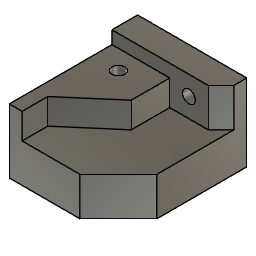
Robocon Task 1-1 (Autodesk Fusion 360 design; units mm, degrees)
Autodesk Fusion 360 part; units mm, degrees
sketch "Sketch1" plane through (0, 0, 0) normal (0, 0, 1) x (1, 0, 0)
  line L0 (0, 0) -> (55, 0)
  line L1 (0, 0) -> (0, 100)
  line L2 (0, 100) -> (85, 100)
  line L3 (85, 100) -> (85, 30)
  line L4 (85, 30) -> (55, 0)
  dimension "d1" = 55
  dimension "d2" = 100
  dimension "d3" = 85
  dimension "d4" = 70
  constraint coincident L0.start L1.start
  constraint horizontal L0
  constraint perpendicular L0 L1
  constraint perpendicular L1 L2
  constraint perpendicular L2 L3
  measures "d1" distance of L0.start L0.end
  measures "d2" distance of L0.start L1.end
  measures "d3" distance of L1.end L2.end
  measures "d4" distance of L2.end L3.end
extrude "Extrude1" add sketch "Sketch1" along normal blind 30
sketch "Sketch2" plane through (0, 0, 30) normal (0, 0, 1) x (-1, 0, 0)
  line L0 (0, 0) -> (-55, 0)
  line L1 (-55, 0) -> (-85, -30)
  line L2 (-85, -30) -> (-85, -100)
  line L3 (-85, -100) -> (0, -100)
  line L4 (0, -100) -> (0, 0)
  line L5 (0, 0) -> (-10, 0)
  line L6 (-10, 0) -> (-10, -20)
  line L7 (0, 0) -> (0, -100)
  line L8 (-85, -100) -> (-85, -90)
  line L9 (-85, -90) -> (-75, -80)
  line L10 (-75, -80) -> (-45, -80)
  line L11 (-45, -80) -> (-45, -50)
  line L12 (-45, -50) -> (-10, -20)
  dimension "d7" = 10
  dimension "d8" = 20
  dimension "d12" = 30
  dimension "d13" = 30
  constraint coincident L0.start L4.end
  constraint perpendicular L4 L5
  constraint perpendicular L5 L6
  constraint coincident L3.end L4.start
  constraint coincident L2.end L3.start
  constraint perpendicular L3 L8
  constraint horizontal L10
  constraint perpendicular L10 L11
  measures "d7" distance of L0.start L5.end
  measures "d8" distance of L5.end L6.end
  measures "d12" distance of L9.end L10.end
  measures "d13" distance of L10.end L11.end
extrude "Extrude2" add sketch "Sketch2" along normal blind 20 contours L0 L2 L3 L4 L5 L6 L7 L8 L9 L10 L11 L12
sketch "Sketch3" plane through (0, 0, 50) normal (0, 0, 1) x (-1, 0, 0)
  line L0 (-85, -100) -> (0, -100)
  line L1 (0, -100) -> (0, 0)
  line L2 (0, 0) -> (-10, 0)
  line L3 (-10, 0) -> (-10, -20)
  line L4 (-10, -20) -> (-45, -50)
  line L5 (-45, -50) -> (-45, -80)
  line L6 (-45, -80) -> (-75, -80)
  line L7 (-75, -80) -> (-85, -90)
  line L8 (-85, -90) -> (-85, -100)
  line L9 (0, -100) -> (0, -80)
  line L10 (0, -80) -> (-75, -80)
  line L11 (-75, -80) -> (-85, -90)
  line L12 (-85, -90) -> (-85, -100)
  line L13 (-85, -100) -> (0, -100)
  dimension "d16" = 20
  constraint coincident L0.end L1.start
  constraint perpendicular L0 L9
  constraint coincident L6.end L7.start
  constraint coincident L7.end L8.start
  constraint coincident L0.start L8.end
  measures "d16" distance of L0.end L9.end
extrude "Extrude3" add sketch "Sketch3" along normal blind 10 contours L0 L1 L6 L7 L8 L9 L10 L11 L12 L13
sketch "Sketch4" plane through (0, 0, 50) normal (0, 0, 1) x (-1, 0, 0)
  line L0 (-45, -80) -> (0, -80)
  line L1 (0, -80) -> (0, 0)
  line L2 (0, 0) -> (-10, 0)
  line L3 (-10, 0) -> (-10, -20)
  line L4 (-10, -20) -> (-45, -50)
  line L5 (-45, -50) -> (-45, -80)
  line L6 (0, -80) -> (0, -65)
  line L7 (0, -65) -> (-20, -65)
  dimension "d20" = 20
  constraint coincident L0.end L1.start
  constraint perpendicular L0 L6
  constraint perpendicular L1 L7
  measures "d20" distance of L6.end L7.end
hole "Hole1" at (20, 65, 50) direction (0, 0, -1) diameter 10 depth 50 tip angle 118
sketch "Sketch5" plane through (0, 80, 0) normal (0, -1, 0) x (1, 0, 0)
  line L0 (45, 30) -> (75, 30)
  line L1 (75, 30) -> (75, 60)
  line L2 (75, 60) -> (0, 60)
  line L3 (0, 60) -> (0, 50)
  line L4 (0, 50) -> (45, 50)
  line L5 (45, 50) -> (45, 30)
  line L6 (45, 50) -> (60, 50)
  line L7 (60, 50) -> (60, 45)
  dimension "d24" = 15
  dimension "d25" = 5
  constraint coincident L4.end L5.start
  constraint perpendicular L5 L6
  constraint perpendicular L0 L7
  measures "d24" distance of L4.end L6.end
  measures "d25" distance of L6.end L7.end
hole "Hole2" at (60, 80, 45) direction (0, 1, 0) diameter 10 depth 20 tip angle 118
